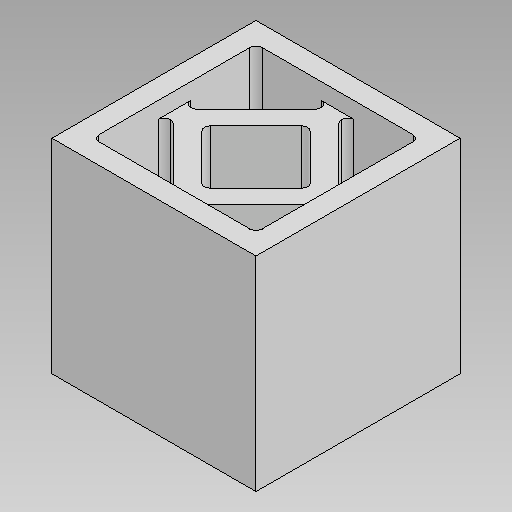
# Autodesk Inventor part: Axle beam base
Saved by Autodesk Inventor 2020 (Build 240168000, 168)
## iProperties
Created: 2019-05-06
Part Number: Axle beam base
Material: Generic
Document SubType Name: Modeling
Designer: Varga Daniel
Density: 1 g/cm^3
Appearance: Default
Author: Varga Daniel
Autodesk Inventor part; units mm, degrees
ref_plane "YZ Plane" through (0, 0, 0) normal (1, 0, 0) x (0, 1, 0)
ref_plane "XZ Plane" through (0, 0, 0) normal (0, 1, 0) x (-1, 0, 0)
ref_plane "XY Plane" through (0, 0, 0) normal (0, 0, 1) x (1, 0, 0)
derived "Base_part.ipt"
sketch "Beam_sketch" plane through (0, 0, 0) normal (0, 1, 0) x (-1, 0, 0)
  circle A0 centre (0, 0) radius 2.5
  line L0 (0, 0) -> (0, -5.5751) construction
  line L1 (3.6649, 0) -> (-4.8297, 0) construction
  arc A1 (-5, 0) -> (0, -5) centre (0, 0) ccw
  line L2 (0, -5) -> (5, -5)
  line L3 (-5, 0) -> (-5, 5)
  line L4 (-5, 5) -> (5, 5)
  line L5 (5, 5) -> (5, -5)
  line L6 (0.5, -3.4641) -> (0.5, -4)
  line L7 (-0.5, -3.2619) -> (-0.5, -4)
  line L8 (0.5, 3.4641) -> (0.5, 4)
  line L9 (-0.5, 3.4641) -> (-0.5, 4)
  line L10 (3.4641, -0.5) -> (4, -0.5)
  line L11 (3.4641, 0.5) -> (4, 0.5)
  line L12 (-3.2619, -0.5) -> (-4, -0.5)
  line L13 (-3.4641, 0.5) -> (-4, 0.5)
  line L14 (-0.5, -4) -> (4, -4)
  arc A2 (-0.5, 3.4641) -> (-3.4641, 0.5) centre (0, 0) ccw
  arc A3 (-3.2619, -0.5) -> (-0.5, -3.2619) centre (0, 0) ccw
  arc A4 (-4.1701, -0.5) -> (-0.5, -4.1701) centre (0, 0) ccw
  line L15 (4, -4) -> (4, -0.5)
  line L16 (4, -0.5) -> (4, 4)
  line L17 (4, 4) -> (0.5, 4)
  line L18 (0.5, 4) -> (-4, 4)
  line L19 (-4, 4) -> (-4, -0.5)
  arc A5 (0.5, -3.4641) -> (3.4641, -0.5) centre (0, 0) ccw
  arc A6 (3.4641, 0.5) -> (0.5, 3.4641) centre (0, 0) ccw
  line L20 (-4, -0.5) -> (-4.1701, -0.5)
  line L21 (-0.5, -4) -> (-0.5, -4.1701)
sketch "Axle_hole_sketch" plane through (0, 0, 0) normal (0, 1, 0) x (-1, 0, 0)
  line L0 (1.575, -1.875) -> (-1.575, -1.875)
  line L1 (-1.875, -1.575) -> (-1.875, 1.575)
  line L2 (-1.575, 1.875) -> (1.575, 1.875)
  line L3 (1.875, 1.575) -> (1.875, -1.575)
  line L4 (1.875, -1.875) -> (-1.875, 1.875) construction
  line L5 (-1.875, -1.875) -> (1.875, 1.875) construction
  arc A0 (1.575, -1.875) -> (1.875, -1.575) centre (1.575, -1.575) ccw
  arc A1 (-1.875, -1.575) -> (-1.575, -1.875) centre (-1.575, -1.575) ccw
  arc A2 (-1.575, 1.875) -> (-1.875, 1.575) centre (-1.575, 1.575) ccw
  arc A3 (1.875, 1.575) -> (1.575, 1.875) centre (1.575, 1.575) ccw
  point P0 (0, 0)
  point P1 (0, 0)
sketch "Sketch3" plane through (0, 0, 0) normal (0, 1, 0) x (-1, 0, 0)
  line L0 (3.6649, 0) -> (-4.8297, 0) construction
  line L1 (0, 0) -> (0, -5.5751) construction
  line L2 (-2.4395, 0.2121) -> (-0.2121, 2.4395)
  line L3 (0.2121, 2.4395) -> (2.4395, 0.2121)
  line L4 (2.4395, -0.2121) -> (0.2121, -2.4395)
  line L5 (-0.2121, -2.4395) -> (-2.4395, -0.2121)
  line L6 (-2.6517, 0) -> (2.6517, 0) construction
  line L7 (0, 2.6517) -> (0, -2.6517) construction
  arc A0 (2.4395, -0.2121) -> (2.4395, 0.2121) centre (2.2274, 0) ccw
  arc A1 (-0.2121, -2.4395) -> (0.2121, -2.4395) centre (0, -2.2274) ccw
  arc A2 (-2.4395, 0.2121) -> (-2.4395, -0.2121) centre (-2.2274, 0) ccw
  arc A3 (0.2121, 2.4395) -> (-0.2121, 2.4395) centre (0, 2.2274) ccw
  line L8 (5, 5) -> (-5, 5)
  line L9 (-5, 5) -> (-5, -5)
  line L10 (-5, -5) -> (5, -5)
  line L11 (5, -5) -> (5, 5)
  line L12 (5, 5) -> (-5, -5) construction
  line L13 (-5, 5) -> (5, -5) construction
  line L14 (4, 4) -> (-4, 4)
  line L15 (-4, 4) -> (-4, -4)
  line L16 (-4, -4) -> (4, -4)
  line L17 (4, -4) -> (4, 4)
  line L18 (4, 4) -> (-4, -4) construction
  line L19 (-4, 4) -> (4, -4) construction
  line L20 (3.5659, 0.5) -> (0.5, 3.5659)
  arc A4 (0.9192, 3.1466) -> (-0.9192, 3.1466) centre (0, 2.2274) ccw
  line L21 (-0.5, 3.5659) -> (-3.5659, 0.5)
  arc A5 (-3.1466, 0.9192) -> (-3.1466, -0.9192) centre (-2.2274, 0) ccw
  line L22 (-3.5659, -0.5) -> (-0.5, -3.5659)
  arc A6 (-0.9192, -3.1466) -> (0.9192, -3.1466) centre (0, -2.2274) ccw
  line L23 (0.5, -3.5659) -> (3.5659, -0.5)
  arc A7 (3.1466, -0.9192) -> (3.1466, 0.9192) centre (2.2274, 0) ccw
  line L24 (0.5, 4) -> (-0.5, 4)
  line L25 (-0.5, 4) -> (-0.5, -4)
  line L26 (-0.5, -4) -> (0.5, -4)
  line L27 (0.5, -4) -> (0.5, 4)
  line L28 (0.5, 4) -> (-0.5, -4) construction
  line L29 (-0.5, 4) -> (0.5, -4) construction
  line L30 (-4, -0.5) -> (4, -0.5)
  line L31 (4, -0.5) -> (4, 0.5)
  line L32 (4, 0.5) -> (-4, 0.5)
  line L33 (-4, 0.5) -> (-4, -0.5)
  line L34 (-4, -0.5) -> (4, 0.5) construction
  line L35 (4, -0.5) -> (-4, 0.5) construction
  point P0 (0, 0)
  point P1 (0, 0)
  point P2 (-0.5, 3.4274)
  point P3 (-3.4274, 0.5)
  point P4 (-3.4274, -0.5)
  point P5 (-0.5, -3.4274)
  point P6 (0.5, -3.4274)
  point P7 (3.4274, -0.5)
  point P8 (3.4274, 0.5)
  point P9 (0.5, 3.4274)
  dimension "d1" = 3.75
  dimension "d2" = 3.75
  dimension "d3" = 0.3
  dimension "d4" = 10
  dimension "d5" = 10
  dimension "d6" = 1
  dimension "d7" = 1
  dimension "d8" = 1
  dimension "d9" = 1
  dimension "d16" = 1
  dimension "d17" = 1
  dimension "d18" = 1
  constraints: 68 end point, 26 point on line, 16 point on circle, 13 midpoint, 13 parallel, 12 tangent, 8 centre point, 6 perpendicular, 4 horizontal, 3 equal radius, 2 collinear
  measures "d1" distance between parallel lines of L2 L4
  measures "d2" distance between parallel lines of L5 L3
  measures "d3" radius of A0
  measures "d4" distance between parallel lines of L9 L11
  measures "d5" distance between parallel lines of L8 L10
  measures "d6" distance between parallel lines of L17 L11
  measures "d7" distance between parallel lines of L3 L20
  measures "d8" distance between parallel lines of L25 L27
  measures "d9" distance between parallel lines of L30 L32
  measures "d16" distance between parallel lines of L22 L5
  measures "d17" distance between parallel lines of L23 L4
  measures "d18" distance between parallel lines of L21 L2
extrude "Extrusion1" add sketch "Sketch3" along normal mid plane 10
extrude "Extrusion2" add sketch "Sketch3" along normal mid plane 8.4 contours A2 L5 L30 A5 L32 L2 | L32 A5 L21 A4 L25 L2 | L25 A4 L27 L3 A3 L2 | L32 L21 A5 | A5 L30 L15 L32 | L5 L25 A6 L22 A5 L30 | L25 L14 L27 A4 | A4 L21 L25 | A5 L22 L30 | L5 A1 L4 L27 A6 L25 | L27 L20 A4 | A4 L20 A7 L32 L3 L27 | L32 A7 L30 L4 A0 L3 | L25 L22 A6 | A6 L27 L16 L25 | L4 L30 A7 L23 A6 L27 | L32 L17 L30 A7 | A7 L20 L32 | A6 L23 L27 | L30 L23 A7
extrude "Extrusion3" add sketch "Sketch3" against normal mid plane 1 contours L32 L21 A5 | A4 L21 L25 | L21 L32 L15 L14 L25 | A5 L22 L30 | L27 L20 A4 | L22 L25 L16 L15 L30 | L25 L22 A6 | L20 L27 L14 L17 L32 | A7 L20 L32 | A6 L23 L27 | L30 L23 A7 | L23 L30 L17 L16 L27
fillet "Fillet1" radius 0.3 32 edges at (3.5659, -2.35, -0.5) (4, -2.35, -0.5) (3.5659, -2.35, 0.5) (4, -2.35, 0.5) (-0.5, -2.35, -4) (-0.5, -2.35, -3.5659) (0.5, -2.35, 3.5659) (0.5, -2.35, 4) (-3.5659, -2.35, -0.5) (-4, -2.35, -0.5) (0.5, -2.35, -4) (0.5, -2.35, -3.5659) (-3.5659, -2.35, 0.5) (-4, -2.35, 0.5) (-0.5, -2.35, 4) (-0.5, -2.35, 3.5659) (0.5, 2.35, 3.5659) (0.5, 2.35, 4) (-0.5, 2.35, 3.5659) (-0.5, 2.35, 4) (-3.5659, 2.35, 0.5) (-4, 2.35, 0.5) (-4, 2.35, -0.5) (-3.5659, 2.35, -0.5) (-0.5, 2.35, -4) (-0.5, 2.35, -3.5659) (0.5, 2.35, -4) (0.5, 2.35, -3.5659) (4, 2.35, -0.5) (3.5659, 2.35, -0.5) (3.5659, 2.35, 0.5) (4, 2.35, 0.5)
fillet "Fillet2" radius 0.3 8 edges at (-4, 2.75, 4) (-4, 2.75, -4) (4, 2.75, 4) (4, 2.75, -4) (4, -2.75, -4) (4, -2.75, 4) (-4, -2.75, 4) (-4, -2.75, -4)
equation "\"d1\" = Axle_hole_width"
equation "\"d2\" = Axle_hole_width"
equation "\"d3\" = Axle_hole_fillet"
equation "\"d4\" = Outer_width"
equation "\"d5\" = Outer_width"
equation "\"d6\" = Wall_thickness"
equation "\"d7\" = Inner_route_thickness"
equation "\"d8\" = Inner_route_thickness"
equation "\"d9\" = Inner_route_thickness"
equation "\"d16\" = Inner_route_thickness"
equation "\"d17\" = Inner_route_thickness"
equation "\"d18\" = Inner_route_thickness"
equation "\"d10\" = Overall_height"
equation "\"d12\" = Hole_height"
equation "\"d14\" = Inner_height"
equation "\"d19\" = Inner_fillet"
equation "\"d20\" = Inner_fillet"
equation "\"Axle_hole_width\" = 3.75"
equation "\"Axle_hole_fillet\" = 0.3"
equation "\"Outer_width\" = 10"
equation "\"Wall_thickness\" = 1"
equation "\"Inner_route_thickness\" = 1"
equation "\"Overall_height\" = 10"
equation "\"Hole_height\" = 8.4"
equation "\"Inner_height\" = 1"
equation "\"Inner_fillet\" = 0.3"
body "Solid1"
